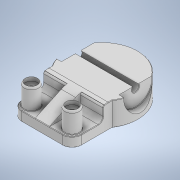
# Autodesk Inventor part: New_Body_Frame
Saved by Autodesk Inventor 2021 (Build 250183000, 183)
## iProperties
Created: 2021-07-26
Part Number: New_Body_Frame
Material: Generic
Document SubType Name: Modeling
Designer: hp
Density: 1 g/cm^3
Appearance: Default
Author: hp
Autodesk Inventor part; units mm, degrees
sketch "Sketch1" plane through (0, 0, 0) normal (0, 1, 0) x (-1, 0, 0)
  circle A0 centre (0, 0) radius 15
  line L0 (12.5, 25) -> (-12.5, 25)
  line L1 (-12.5, 25) -> (-12.5, 5)
  line L2 (-12.5, 5) -> (12.5, 5)
  line L3 (12.5, 5) -> (12.5, 25)
  line L4 (12.5, 25) -> (-12.5, 5) construction
  line L5 (-12.5, 25) -> (12.5, 5) construction
  point P0 (0, 15)
  point P1 (-12.5, 8.2916)
  point P2 (12.5, 8.2916)
  dimension "d0" = 30
  dimension "d1" = 25
  dimension "d2" = 20
  constraints: 12 end point, 2 midpoint, 2 parallel, 1 coincident, 1 horizontal, 1 perpendicular, 3 other
  measures "d1" distance of L2.end L1.end
  measures "d2" distance of L0.end L1.end
extrude "Extrusion1" add sketch "Sketch1" along normal blind 10
ref_plane "Work Plane1" through (15, 0, 0) normal (1, 0, 0) x (0, 1, 0)
sketch "Sketch2" plane through (15, 0, 0) normal (1, 0, 0) x (0, 1, 0)
  line L0 (0, 0) -> (9, 0)
  line L1 (9, 0) -> (9, -2)
  circle A0 centre (9, -2) radius 7
  dimension "d7" = 9
  dimension "d8" = 2
  dimension "d9" = 14
  constraints: 4 end point, 1 centre point, 1 coincident, 1 horizontal, 1 vertical
  measures "d7" distance of L0.start L0.end
  measures "d8" distance of L0.end L1.end
  measures "d9" diameter of A0
extrude "Extrusion2" cut sketch "Sketch2" against normal blind 3
ref_plane "Work Plane2" through (-15, 0, 0) normal (1, 0, 0) x (0, 1, 0)
sketch "Sketch3" plane through (-15, 0, 0) normal (1, 0, 0) x (0, 1, 0)
  line L0 (0, 0) -> (9, 0)
  line L1 (9, 0) -> (9, -2)
  circle A0 centre (9, -2) radius 7
  dimension "d13" = 9
  dimension "d14" = 2
  dimension "d15" = 14
  constraints: 4 end point, 1 centre point, 1 coincident, 1 horizontal, 1 perpendicular
  measures "d13" distance of L0.start L0.end
  measures "d14" distance of L0.end L1.end
  measures "d15" diameter of A0
extrude "Extrusion3" cut sketch "Sketch3" along normal blind 3
sketch "Sketch4" plane through (0, 0, 0) normal (1, 0, 0) x (0, 1, 0)
  line L0 (0, 0) -> (9, 0)
  line L1 (9, 0) -> (9, -2)
  circle A0 centre (9, -2) radius 1.5
  line L2 (0, 0) -> (0, 12)
  line L3 (0, 12) -> (10, 12)
  line L4 (10, 8.2916) -> (10, 25) projected
  line L5 (0, 25) -> (10, 25) projected
  line L6 (10, 12) -> (4, 12)
  line L7 (4, 12) -> (4, 25)
  line L8 (4, 25) -> (10, 25)
  line L9 (10, 25) -> (10, 12)
  line L10 (4, 25) -> (10, 12)
  dimension "d18" = 9
  dimension "d19" = 2
  dimension "d20" = 3
  dimension "d21" = 12
  dimension "d22" = 6
  constraints: 18 end point, 3 horizontal, 3 perpendicular, 2 parallel, 2 point on line, 1 centre point, 1 coincident
  measures "d18" distance of L0.start L0.end
  measures "d19" distance of L0.end L1.end
  measures "d20" diameter of A0
  measures "d21" distance of L0.start L2.end
  measures "d22" distance of L7.end L8.end
extrude "Extrusion4" cut sketch "Sketch4" against normal through all both and the other way through all contours A0 | L10 L5 L4
sketch "Sketch5" plane through (15, 0, 0) normal (1, 0, 0) x (0, 1, 0)
  line L0 (0, 25) -> (4, 25) projected
  line L1 (10, 12) -> (10, 8.2916) projected
  line L2 (4, 25) -> (10, 25)
  line L3 (10, 25) -> (10, 12)
  line L4 (10, 12) -> (4, 12)
  line L5 (4, 12) -> (4, 25)
  point P0 (0, 0)
  constraints: 8 end point, 2 parallel, 1 horizontal, 1 perpendicular
extrude "Extrusion5" cut sketch "Sketch5" against normal blind 12
sketch "Sketch6" plane through (-15, 0, 0) normal (1, 0, 0) x (0, 1, 0)
  line L0 (10, 8.2916) -> (10, 12) projected
  line L1 (4, 25) -> (10, 25)
  line L2 (10, 25) -> (10, 12)
  line L3 (10, 12) -> (4, 12)
  line L4 (4, 12) -> (4, 25)
  point P0 (0, 0)
  constraints: 8 end point, 2 parallel, 1 horizontal, 1 perpendicular
extrude "Extrusion6" cut sketch "Sketch6" along normal blind 12
ref_plane "Work Plane3" through (-12.5, 4, 25) normal (0, 1, 0) x (1, 0, 0)
sketch "Sketch7" plane through (-12.5, 4, 25) normal (0, 1, 0) x (1, 0, 0)
  line L0 (9.5, 0) -> (0, 0) projected
  line L1 (0, 0) -> (4, 0)
  line L2 (4, 0) -> (4, 4)
  circle A0 centre (4, 4) radius 3
  line L3 (25, 0) -> (21, 0)
  line L4 (0, 0) -> (25, 0) projected
  line L5 (21, 0) -> (21, 4)
  circle A1 centre (21, 4) radius 3
  point P0 (12.5, 25)
  dimension "d30" = 4
  dimension "d31" = 4
  dimension "d32" = 6
  dimension "d33" = 4
  dimension "d34" = 4
  dimension "d35" = 6
  constraints: 8 end point, 2 centre point, 2 coincident, 2 perpendicular, 2 point on line
  measures "d30" distance of L0.end L1.end
  measures "d31" distance of L1.end L2.end
  measures "d32" diameter of A0
  measures "d33" distance of L3.start L3.end
  measures "d34" distance of L3.end L5.end
  measures "d35" diameter of A1
extrude "Extrusion7" add sketch "Sketch7" along normal blind 8.6
sketch "Sketch8" plane through (-12.5, 4, 25) normal (0, 1, 0) x (1, 0, 0)
  circle A0 centre (4, 4) radius 3 projected
  circle A1 centre (4, 4) radius 4
  line L0 (0, 0) -> (25, 0) projected
  line L1 (4, 4) -> (0, 4)
  line L2 (0, 4) -> (0, 0)
  line L3 (0, 0) -> (4, 0)
  line L4 (4, 0) -> (4, 4)
  circle A2 centre (21, 4) radius 3 projected
  line L5 (21, 4) -> (25, 4)
  line L6 (25, 4) -> (25, 0)
  line L7 (25, 0) -> (21, 0)
  line L8 (21, 0) -> (21, 4)
  circle A3 centre (21, 4) radius 4
  point P0 (12.5, 25)
  point P1 (4, 0)
  constraints: 16 end point, 4 parallel, 2 coincident, 2 horizontal, 2 perpendicular, 1 centre point, 1 tangent, 3 other
extrude "Extrusion8" cut sketch "Sketch8" against normal blind 8.6 contours A1 L0 L2 | A3 L6 L0
ref_plane "Work Plane4" through (-8.5, 12.6, 21) normal (0, 1, 0) x (1, 0, 0)
sketch "Sketch9" plane through (-8.5, 12.6, 21) normal (0, 1, 0) x (1, 0, 0)
  circle A0 centre (17, 0) radius 3 projected
  circle A1 centre (17, 0) radius 2.5
  circle A2 centre (0, 0) radius 2.5
  point P0 (8.5, 21)
  dimension "d41" = 5
  dimension "d42" = 5
  constraints: 2 centre point, 1 coincident
  measures "d41" diameter of A1
  measures "d42" diameter of A2
extrude "Extrusion9" cut sketch "Sketch9" against normal blind 2.6 contours A1 | A2
fillet "Fillet1" radius 1 4 edges at (5.5, 12.6, 21) (-11.5, 12.6, 21) (-11, 10, 21) (6, 10, 21)
fillet "Fillet2" radius 2 2 edges at (-7.75, 4, 12) (7.75, 4, 12)
fillet "Fillet3" radius 1 2 edges at (7.75, 10, 12) (-7.75, 10, 12)
fillet "Fillet4" radius 10 1 edges at (0, 10, 12)
fillet "Fillet5" radius 0.2 17 edges at (11.3284, 0, 23.8284) (12.5, 0, 14.6458) (-11.3284, 0, 23.8284) (-12.5, 0, 14.6458) (0, 0, 25) (0, 0, -15) (12, 2.018, -1.4987) (12, 7.5, -2) (-12, 2.018, -1.4987) (-12, 7.5, -2) (0, 10, -15) (-13.4393, 10, 6.6622) (-12.5, 9.9626, 10.668) (-12.5, 10, 9.0476) (13.4393, 10, 6.6622) (12.5, 10, 9.0476) (12.5, 9.9626, 10.668)
fillet "Fillet6" radius 0.2 2 edges at (-11.5, 4, 21) (5.5, 4, 21)
sketch "Sketch10" plane through (0, 0, 0) normal (0, 1, 0) x (-1, 0, 0)
  circle A0 centre (0, 0) radius 5
  dimension "d51" = 10
  constraints: 1 centre point, 1 coincident
  measures "d51" diameter of A0
extrude "Extrusion10" add sketch "Sketch10" against normal blind 1
fillet "Fillet7" radius 0.2 2 edges at (5, 0, 0) (5, -1, 0)
fillet "Fillet8" radius 0.2 16 edges at (-12.5, 4, 17.5) (-11.3284, 4, 23.8284) (-5.75, 4, 25) (-12.5, 7.5, 12) (-12.5, 9.3124, 11.95) (-12.443, 9.7688, 11.6395) (-7.65, 9.8506, 11.5258) (-12.5, 4.5858, 12.5858) (11.3284, 4, 23.8284) (12.5, 4, 17.5) (12.5, 4.5858, 12.5858) (12.5, 7.5, 12) (12.5, 9.3124, 11.95) (12.443, 9.7688, 11.6395) (7.65, 9.8506, 11.5258) (5.75, 4, 25)
fillet "Fillet9" radius 0.3 1 edges at (0, 4, 25)
body "Solid1"
